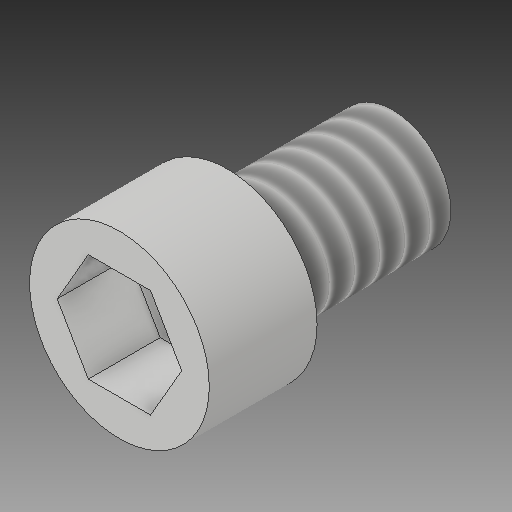
# Autodesk Inventor part: M4 sujecion
Saved by Autodesk Inventor 2019.2 (Build 232265000, 265)
## iProperties
Created: 2018-03-09
Part Number: M4 sujecion
Material: Generic
Document SubType Name: Modeling
Designer: Hogar
Density: 1 g/cm^3
Appearance: Default
Author: Hogar
Autodesk Inventor part; units mm, degrees
ref_plane "YZ Plane" through (0, 0, 0) normal (1, 0, 0) x (0, 1, 0)
ref_plane "XZ Plane" through (0, 0, 0) normal (0, 1, 0) x (-1, 0, 0)
ref_plane "XY Plane" through (0, 0, 0) normal (0, 0, 1) x (1, 0, 0)
sketch "Sketch1" plane through (0, 0, 0) normal (0, 0, 1) x (1, 0, 0)
  circle A0 centre (0, 0) radius 1.621
  dimension "d0" = 3.242
  constraints: 1 centre point, 1 coincident
  measures "d0" diameter of A0
extrude "Extrusion1" add sketch "Sketch1" along normal blind 4.6
sketch "Sketch2" plane through (0, 0, 4.6) normal (0, 0, 1) x (1, 0, 0)
  circle A0 centre (0, 0) radius 2.5
  dimension "d3" = 5
  constraints: 1 centre point, 1 coincident
  measures "d3" diameter of A0
extrude "Extrusion2" add sketch "Sketch2" along normal blind 3
sketch "Sketch3" plane through (0, 0, 7.6) normal (0, 0, 1) x (1, 0, 0)
  line L0 (0.866, 1.5) -> (1.7321, 0)
  line L1 (1.7321, 0) -> (0.866, -1.5)
  line L2 (0.866, -1.5) -> (-0.866, -1.5)
  line L3 (-0.866, -1.5) -> (-1.7321, 0)
  line L4 (-1.7321, 0) -> (-0.866, 1.5)
  line L5 (-0.866, 1.5) -> (0.866, 1.5)
  point P0 (0, 0)
  dimension "d14" = 3
  constraints: 12 end point, 13 other
  measures "d14" distance between parallel lines of L2 L5
extrude "Extrusion3" cut sketch "Sketch3" against normal blind 2
thread "Thread1" size "M4x0.7" class "6g" standard "ANSI Metric M Profile" full length
body "Solid1"
